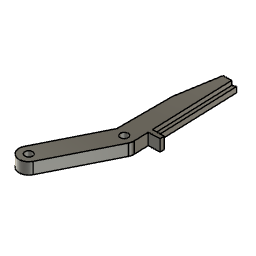
_ConnectorArmV2.a69f7e0e-7f39-4681-87bd-2c2f9123c0e2 (Autodesk Fusion 360 design; units mm, degrees)
Autodesk Fusion 360 part; units mm, degrees
other "Derived from MasterParameters_Gripper v58"
sketch "Sketch1" plane through (0, 0, 0) normal (0, 0, 1) x (1, 0, 0)
  circle A0 centre (0, 0) radius 3.35
  circle A1 centre (-11, -22) radius 3.35
  circle A2 centre (-11, -22) radius 1.35
  circle A3 centre (0, 0) radius 1.35
  line L0 (2.9963, -1.4982) -> (-8.0037, -23.4982)
  line L1 (-2.9963, 1.4982) -> (-13.9963, -20.5018)
  line L2 (3.35, 0.0611) -> (2.0883, 35.1057)
  line L3 (2.0883, 35.1057) -> (-0.8471, 35)
  line L4 (-0.8471, 35) -> (-3.35, 20)
  line L5 (-3.35, 0) -> (-3.35, 20)
  constraint coincident A0.centre A3.centre
  constraint concentric A1 A2
  constraint equal A2 A3
  constraint equal A0 A1
  constraint coincident A0 L0.start
  constraint coincident A1 L0.end
  constraint tangent A1 L0
  constraint coincident A1 L1.end
  constraint tangent A1 L1
  constraint tangent A0 L0
  constraint perpendicular L2 L3
  constraint tangent A0 L2
  constraint tangent A0 L1
  constraint vertical L5
  constraint tangent A0 L5
  constraint coincident A0 L5.start
  measures "d1" distance of A0.centre A1.centre
  measures "d30" diameter of A3
  measures "d31" distance of A1 A2
  measures "d32" distance of A1.centre A0.centre
  measures "d54" distance of L5.start L4.end
  measures "d59" distance of L3.end L4.end
extrude "Extrude1" add sketch "Sketch1" along normal blind 4
sketch "Sketch3" plane through (-1.2596, 34.9851, 0) normal (-0.03598, 0.999353, 0) x (-0.999353, -0.03598, 0)
  line L0 (-3.35, 0) -> (-0.4128, 0)
  line L1 (-0.4128, 0) -> (-0.4128, 4)
  line L2 (-0.4128, 4) -> (-3.35, 4)
  line L3 (-3.35, 4) -> (-3.35, 0)
  line L4 (-3.35, 2) -> (-4.9507, 2) construction
  line L5 (-4.9507, 1.065) -> (-4.9507, 2.935)
  line L6 (-4.9507, 2.935) -> (-3.35, 2.4949)
  line L7 (-4.9507, 1.065) -> (-3.35, 1.5051)
  constraint midpoint L3 L4.start
  constraint perpendicular L3 L4
  constraint perpendicular L4 L5
  constraint coincident L4.end L5
  constraint midpoint L4.end L5
  constraint coincident L3 L6.end
  constraint symmetric L4 L5.end L5.start
  constraint symmetric L4 L6.end L7.end
sketch "Sketch4" plane through (3.3478, 0.1205, 0) normal (0.999353, 0.03598, 0) x (-0.03598, 0.999353, 0)
  line L0 (35.0078, 0) -> (35.0078, 4)
  line L1 (35.0078, 4) -> (0, 4)
  line L2 (0, 4) -> (0, 0)
  line L3 (0, 0) -> (35.0078, 0)
  line L4 (5, 4) -> (6.5, 4)
  line L5 (6.5, 4) -> (6.5, 0)
  line L6 (6.5, 0) -> (5, 0)
  line L7 (5, 0) -> (5, 4)
  line L8 (0, 4) -> (35.0078, 4)
  line L9 (0, 0) -> (35.0078, 0)
  dimension "d48" = 1.5
  dimension "d55" = 5
  constraint horizontal L4
  constraint vertical L5
  constraint horizontal L6
  constraint vertical L7
  constraint coincident L3 L5.end
  constraint coincident L4.start L7.end
  constraint coincident L1 L4.start
  measures "d48" distance of L5 L7
  measures "d55" distance of L2 L7
extrude "Extrude3" add sketch "Sketch4" along normal blind 4 contours L1 L3 L4 L5 L6 L7 L8 L9
extrude "Extrude4" add sketch "Sketch3" against normal up to surface (28.5078 mm away) contours L3 L5 L6 L7
equation "d1 = plate_distance_back_front_y_Ref"
equation "m2_nut_diameter_Ref = 4.2 mm"
equation "m2_nut_height_Ref = 3 mm"
equation "arm_screw_wall_thickness_Ref = 1 mm"
equation "m2_screw_diameter_Ref = 2.2 mm" comment "diameter with tolerance"
equation "m25_screw_diameter_Ref = 2.7 mm"
equation "m25_wall_thickness_Ref = 2 mm"
equation "m2_tapping_tolerance_Ref = 0.2 mm"
equation "Servo_cut_gap_Ref = 0.5 mm"
equation "m25_screw_head_height_Ref = 2.5 mm"
equation "m25_screw_head_width_Ref = 4.6 mm"
equation "m25_arm_screw_plus_tolerance_Ref = 2.9 mm" comment "Additional parameter to experiment with parameter to hopefully enable free movement of arm"
equation "m2_tapping_head_width_Ref = 4 mm"
equation "back_arms_thickness_Ref = 8 mm"
equation "m2_screw_head_diameter_Ref = 4 mm"
equation "m2_screw_head_height_Ref = 2 mm"
equation "arm_height_Ref = 4 mm"
equation "arm_ground_clearance_Ref = 1 mm"
equation "m3_screw_diameter_Ref = 3.2 mm"
equation "m3_wall_thickness_gripper_mount_Ref = 2 mm"
equation "arm_length_Ref = 25 mm"
equation "gear_arm_gap_Ref = 0.05 mm"
equation "distance_lower_upper_plate_Ref = 10 mm"
equation "gear_screw_dist_Ref = 1.5 mm"
equation "gear_z_height_placement_on_arm_Ref = 5 mm"
equation "plate_distance_back_axes_Ref = 30 mm" comment "Distance between back-axes, namely servo and the arm axis of the arm in the back"
equation "plate_distance_back_front_x_Ref = 11 mm" comment "Distance from the back to the front axis"
equation "d30 = m25_screw_diameter_Ref"
equation "d31 = m25_wall_thickness_Ref"
equation "d32 = plate_distance_back_front_x_Ref"
equation "d33 = arm_height_Ref"
equation "gear_arm_connector_height_Ref = 4 mm"
equation "m25_ruthex_outer_Ref = 7.2 mm"
equation "m25_ruthex_inner_Ref = 4 mm"
equation "m25_ruthex_height_Ref = 5.7 mm"
equation "plate_single_height_Ref = 3 mm" comment "height of a single plate piece"
equation "plate_distance_back_front_y_Ref = 22 mm"
equation "stand_width_Ref = 5 mm" comment "width of the stand that the gripper can be mounted onto"
equation "gripper_tpu_thickness_Ref = 4 mm"
equation "d53 = gripper_tpu_thickness_Ref"
equation "arm_top_tolerance_Ref = 0.2 mm"
